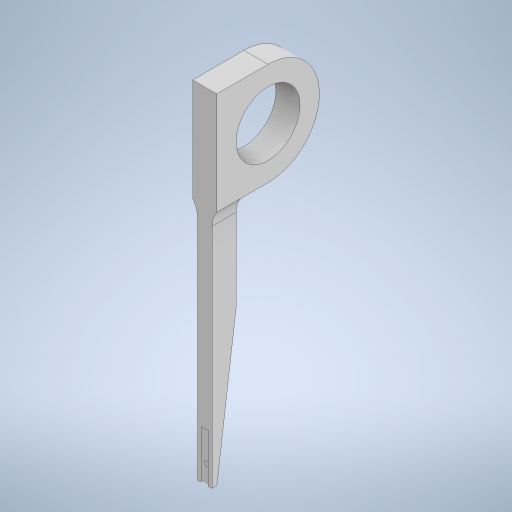
# Autodesk Inventor part: washing_arm
Saved by Autodesk Inventor 2023.3 (Build 273359000, 359)
## iProperties
Created: 2023-11-21
Part Number: washing_arm
Material: Generic
Document SubType Name: Modeling
Designer: mmelin
Density: 1 g/cm^3
Appearance: Default
Author: mmelin
Autodesk Inventor part; units mm, degrees
ref_plane "YZ Plane" through (0, 0, 0) normal (1, 0, 0) x (0, 1, 0)
ref_plane "XZ Plane" through (0, 0, 0) normal (0, 1, 0) x (-1, 0, 0)
ref_plane "XY Plane" through (0, 0, 0) normal (0, 0, 1) x (1, 0, 0)
sketch "Sketch1" plane through (0, 0, 0) normal (1, 0, 0) x (0, 1, 0)
  circle A0 centre (0, 0) radius 6.604
  circle A1 centre (0, 0) radius 10.604
  line L0 (10.604, 0) -> (-10.604, 0)
  line L1 (-10.604, 0) -> (-10.604, 10.604)
  line L2 (-10.604, 10.604) -> (10.604, 10.604)
  line L3 (10.604, 10.604) -> (10.604, 0)
  point P0 (-10.604, 0)
  dimension "d1" = 21.208
  dimension "d0" = 13.208
  constraints: 8 end point, 2 coincident, 2 horizontal, 2 parallel, 2 vertical, 1 centre point, 1 perpendicular, 3 other
  measures "d0" diameter of A0
extrude "Extrusion1" add sketch "Sketch1" along normal blind 5 contours L0 A1 A0 | A0 L0 A1 | A1 L2 L3 | L1 L2 A1
sketch "Sketch2" plane through (0, -10.604, 0) normal (0, -1, 0) x (1, 0, 0)
  line L0 (0, 0) -> (0, 10.604) projected
  line L1 (5, 0) -> (5, 10.604) projected
  line L2 (1, 10.604) -> (4, 10.604)
  line L3 (4, 10.604) -> (4, 5.604)
  line L4 (4, 5.604) -> (1, 5.604)
  line L5 (1, 5.604) -> (1, 10.604)
  line L6 (0, 10.604) -> (5, 10.604) projected
  dimension "d16" = 1
  dimension "d17" = 1
  dimension "d18" = 5
  constraints: 8 end point, 2 parallel, 1 collinear, 1 horizontal, 1 perpendicular
  measures "d16" distance between parallel lines of L1 L3
  measures "d17" distance between parallel lines of L0 L5
  measures "d18" distance between parallel lines of L2 L4
extrude "Extrusion2" add sketch "Sketch2" along normal blind 50
sketch "Sketch3" plane through (0, -60.604, 0) normal (0, -1, 0) x (1, 0, 0)
  line L0 (1.329, 10.154) -> (3.671, 10.154)
  line L1 (1.329, 10.154) -> (1.779, 10.604)
  line L2 (3.671, 10.154) -> (3.221, 10.604)
  line L3 (1.329, 10.154) -> (1.658, 10.154) construction
  line L4 (3.671, 10.154) -> (4, 10.154) construction
  line L5 (4, 10.604) -> (1, 10.604) projected
  line L6 (1.329, 10.154) -> (1, 10.154) construction
  line L7 (1, 10.604) -> (1, 5.604) construction
  line L8 (4, 5.604) -> (4, 10.604) construction
  point P0 (0, 0)
  dimension "d6" = 2.342
  dimension "d7" = 45
  dimension "d8" = 45
  dimension "d19" = 0.45
  constraints: 12 end point, 4 point on line, 3 equal length, 2 horizontal, 1 collinear
  measures "d6" distance of L0.start L0.end
  measures "d7" angle of L0 L1
  measures "d8" angle of L0 L2
  measures "d19" distance between parallel lines of L5 L0
extrude "Extrusion3" cut sketch "Sketch3" against normal blind 10
chamfer "Chamfer1" distance 4 distance2 30 1 edges at (2.5, -60.604, 5.604) measured on face at (2.8903, -60.604, 7.1207)
fillet "Fillet1" radius 5 2 edges at (4, -10.604, 8.104) (1, -10.604, 8.104)
sketch "Sketch4" plane through (1.329, -60.604, 10.154) normal (0, 0, 1) x (1, 0, 0)
  circle A0 centre (1.171, 3.5) radius 0.45
  line L0 (1.171, 3.5) -> (2.671, 3.5) construction
  line L1 (1.171, 3.5) -> (-0.329, 3.5)
  line L2 (-0.329, 47) -> (-0.329, 0) construction
  line L3 (2.671, 47) -> (2.671, 0) construction
  line L4 (2.342, 0) -> (0, 0) construction
  point P0 (-1.329, 60.604)
  dimension "d21" = 0.9
  dimension "d22" = 3.5
  constraints: 4 end point, 2 horizontal, 2 point on line, 1 centre point, 1 collinear, 1 perpendicular
  measures "d21" diameter of A0
  measures "d22" distance from line of L4 L0.start
extrude "Extrusion4" cut sketch "Sketch4" against normal blind 10
sketch "Sketch5" plane through (1.329, -60.604, 10.154) normal (0, 0, 1) x (1, 0, 0)
  circle A0 centre (1.171, 3.5) radius 0.45 projected
  circle A1 centre (1.171, 3.5) radius 0.75
  point P0 (-1.329, 60.604)
  dimension "d25" = 1.5
  constraints: 1 centre point, 1 coincident
  measures "d25" diameter of A1
extrude "Extrusion5" add sketch "Sketch5" against normal blind 1.5
equation "\"d17\" = d16"
equation "\"d8\" = d7"
body "Solid1"
